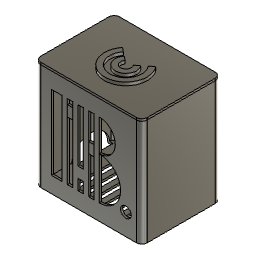
enclosure-lastEdition (Autodesk Fusion 360 design; units mm, degrees)
Autodesk Fusion 360 part; units mm, degrees
note: some values were not read from the file. Chosen so that the rebuilt part matches the saved one: which bodies a step acts on. Set by a fixed rule: which sketch regions a step uses.
sketch "Sketch1" plane through (0, 0, 0) normal (0, 0, 1) x (1, 0, 0)
  line L0 (0, 0) -> (100, 0)
  line L1 (100, 0) -> (100, 74)
  line L2 (100, 74) -> (0, 74)
  line L3 (0, 74) -> (0, 0)
  dimension "d1" = 100
  dimension "d2" = 74
  constraint horizontal L0
  constraint vertical L1
  constraint horizontal L2
  constraint vertical L3
  constraint coincident L0.start L3.end
  measures "d1" distance of L0.start L0.end
  measures "d2" distance of L0.start L2.end
extrude "Extrude1" add sketch "Sketch1" along normal blind 100 makes body 1
fillet "Fillet1" radius 5 1 edges at (100, 0, 50) on bodies 1
fillet "Fillet2" radius 5 1 edges at (0, 0, 50) on bodies 1
fillet "Fillet3" radius 5 1 edges at (100, 74, 50) on bodies 1
fillet "Fillet4" radius 5 1 edges at (0, 74, 50) on bodies 1
shell "Shell1" thickness 2 removed faces 1 at (35, 24.6667, 100) on bodies 1
sketch "Sketch2" plane through (0, 0, 0) normal (-1, 0, 0) x (0, -1, 0)
  line L0 (-69, 100) -> (-69, 0)
  line L1 (-69, 0) -> (-5, 0)
  line L2 (-5, 0) -> (-5, 100)
  line L3 (-5, 100) -> (-69, 100)
  circle A0 centre (-50, 0) radius 18
  dimension "d14" = 36
  constraint coincident L1 A0.centre
  measures "d14" diameter of A0
extrude "Extrude2" cut sketch "Sketch2" against normal blind 5 contours L1 A0 picked at (-55.0244, 4.2742) bodies 1
sketch "Sketch3" plane through (0, 74, 0) normal (0, 1, 0) x (-1, 0, 0)
  line L0 (-5, 0) -> (-5, 100)
  line L1 (-5, 100) -> (-95, 100)
  line L2 (-95, 100) -> (-95, 0)
  line L3 (-95, 0) -> (-5, 0)
  line L4 (-45.9741, 3.8259) -> (-20.9741, 3.8259) construction
  line L5 (-20.9741, 3.8259) -> (-20.9741, 13.8259) construction
  line L6 (-20.9741, 13.8259) -> (-45.9741, 13.8259) construction
  line L7 (-45.9741, 13.8259) -> (-45.9741, 3.8259) construction
  dimension "d17" = 10
  text T0 "CASA" font "Arial" height 10 align left top in box 25 x 10 at (-45.9741, 3.8259) x (1, 0) y (0, 1) spacing 1
extrude "Extrude3" cut sketch "Sketch3" against normal blind 10 text T0 bodies 1 makes body 2 at (13.1683, 72, 8.8554) makes body 3 at (35, 0, 33.3333)
sketch "Sketch4" plane through (0, 0, 0) normal (0, 0, 1) x (1, 0, 0)
sketch "Sketch5" plane through (0, 0, 0) normal (0, 1, 0) x (1, 0, 0)
  line L0 (5, 0) -> (15, 0)
  line L1 (15, -15) -> (25, -15)
  line L2 (25, -15) -> (25, -85)
  line L3 (25, -85) -> (15, -85)
  line L4 (15, -85) -> (15, -15)
  line L5 (30, -15) -> (35, -15)
  line L6 (35, -15) -> (35, -85)
  line L7 (35, -85) -> (30, -85)
  line L8 (30, -85) -> (30, -15)
  line L9 (40, -15) -> (45, -15)
  line L10 (45, -15) -> (45, -85)
  line L11 (45, -85) -> (40, -85)
  line L12 (40, -85) -> (40, -15)
  line L13 (50, -15) -> (55, -15)
  line L14 (55, -15) -> (55, -85)
  line L15 (55, -85) -> (50, -85)
  line L16 (50, -85) -> (50, -15)
  arc A0 (60, -85) -> (60, -55) centre (60, -70) ccw
  arc A1 (60, -55) -> (60, -15) centre (60, -35) ccw
  line L17 (60, -85) -> (60, -15)
  line L18 (40, -25) -> (38, -25)
  line L19 (38, -25) -> (38, -35)
  line L20 (38, -35) -> (40, -35)
  line L21 (40, -35) -> (40, -25)
  line L22 (40, -25) -> (47, -25)
  line L23 (47, -25) -> (47, -35)
  line L24 (47, -35) -> (40, -35)
  line L25 (40, -35) -> (40, -25)
  line L26 (30, -70) -> (28, -70)
  line L27 (28, -80) -> (30, -80)
  line L28 (30, -80) -> (30, -70)
  line L29 (30, -70) -> (37, -70)
  line L30 (37, -80) -> (30, -80)
  line L31 (30, -80) -> (30, -70)
  line L32 (50, -50) -> (48, -50)
  line L33 (48, -50) -> (48, -60)
  line L34 (48, -60) -> (50, -60)
  line L35 (50, -60) -> (50, -50)
  line L36 (48, -50) -> (57, -50)
  line L37 (57, -50) -> (57, -60)
  line L38 (57, -60) -> (48, -60)
  line L39 (48, -60) -> (48, -50)
  dimension "d22" = 2
  dimension "d23" = 10
  dimension "d24" = 7
  dimension "d25" = 10
  dimension "d26" = 2
  dimension "d27" = 7
  dimension "d28" = 2
  dimension "d29" = 9
  dimension "d30" = 10
  constraint horizontal L0
  constraint horizontal L1
  constraint vertical L2
  constraint horizontal L3
  constraint vertical L4
  constraint horizontal L5
  constraint vertical L6
  constraint horizontal L7
  constraint vertical L8
  constraint horizontal L9
  constraint vertical L10
  constraint horizontal L11
  constraint vertical L12
  constraint horizontal L13
  constraint vertical L14
  constraint horizontal L15
  constraint vertical L16
  constraint vertical L17
  constraint horizontal L18
  constraint vertical L19
  constraint horizontal L20
  constraint vertical L21
  constraint coincident L12 L18.start
  constraint horizontal L22
  constraint vertical L23
  constraint horizontal L24
  constraint vertical L25
  constraint horizontal L26
  constraint horizontal L27
  constraint vertical L28
  constraint coincident L8 L26.start
  constraint horizontal L29
  constraint horizontal L30
  constraint vertical L31
  constraint horizontal L32
  constraint vertical L33
  constraint horizontal L34
  constraint vertical L35
  constraint midpoint L16 L32.start
  constraint horizontal L36
  constraint vertical L37
  constraint horizontal L38
  constraint vertical L39
  measures "d22" distance of L18.start L18.end
  measures "d23" distance of L18.start L20.end
  measures "d24" distance of L18.start L22.end
  measures "d25" distance of L18.start L20.end
  measures "d26" distance of L26.start L26.end
  measures "d27" distance of L26.start L29.end
  measures "d28" distance of L32.start L32.end
  measures "d29" distance of L32.end L36.end
  measures "d30" distance of L32.end L33.end
extrude "Extrude5" cut sketch "Sketch5" along normal blind 5 contours L1 L2 L3 L4 bodies 3
extrude "Extrude4" cut sketch "Sketch5" along normal blind 5 contours L1 L2 L3 L4 bodies 3
extrude "Extrude6" cut sketch "Sketch5" along normal blind 5 contours L5 L6 L8 L29 bodies 3
extrude "Extrude7" cut sketch "Sketch5" along normal blind 5 contours L10 L11 L12 L24 bodies 3
extrude "Extrude8" cut sketch "Sketch5" along normal blind 10 contours A1 L17 bodies 3
extrude "Extrude9" cut sketch "Sketch5" along normal blind 5 contours A0 L17 bodies 3
extrude "Extrude10" cut sketch "Sketch5" along normal blind 5 contours L14 L15 L16 L38 bodies 3
extrude "Extrude11" cut sketch "Sketch5" along normal blind 5 contours L13 L14 L16 L36 bodies 3
extrude "Extrude12" cut sketch "Sketch5" along normal blind 5 contours L6 L8 L28 L29 L30 L31 bodies 3
extrude "Extrude13" cut sketch "Sketch5" along normal blind 5 contours L14 L16 L35 L36 L38 bodies 3
extrude "Extrude14" add sketch "Sketch5" along normal blind 2 separate body contours L14 L16 L35 L36 L38 makes body 4
extrude "Extrude15" add sketch "Sketch5" along normal blind 2 separate body contours L6 L8 L28 L29 L30 L31 makes body 5
extrude "Extrude16" cut sketch "Sketch5" along normal blind 2 contours L9 L10 L12 L22 bodies 3
extrude "Extrude17" cut sketch "Sketch5" along normal blind 2 contours L6 L7 L8 L30 bodies 3
sketch "Sketch6" plane through (0, 0, 0) normal (0, -1, 0) x (1, 0, 0)
  line L0 (35, 85) -> (35, 15)
  line L1 (35, 15) -> (30, 15)
  line L2 (30, 15) -> (30, 85)
  line L3 (30, 85) -> (35, 85)
  line L4 (45, 15) -> (40, 15)
  line L5 (40, 15) -> (40, 25)
  line L6 (40, 25) -> (45, 25)
  line L7 (45, 25) -> (45, 15)
  line L8 (50, 15) -> (50, 85)
  line L9 (50, 85) -> (55, 85)
  line L10 (55, 85) -> (55, 15)
  line L11 (55, 15) -> (50, 15)
  line L12 (5, 100) -> (5, 0)
  line L13 (5, 0) -> (95, 0)
  line L14 (95, 0) -> (95, 100)
  line L15 (95, 100) -> (5, 100)
  line L16 (15, 15) -> (15, 85)
  line L17 (15, 85) -> (25, 85)
  line L18 (25, 85) -> (25, 15)
  line L19 (25, 15) -> (15, 15)
  line L20 (45, 85) -> (45, 35)
  line L21 (45, 35) -> (40, 35)
  line L22 (40, 35) -> (40, 85)
  line L23 (40, 85) -> (45, 85)
  line L24 (60, 15) -> (60, 55)
  line L25 (60, 55) -> (60, 85)
  arc A0 (60, 55) -> (60, 85) centre (60, 70) ccw
  arc A1 (60, 15) -> (60, 55) centre (60, 35) ccw
  circle A2 centre (85, 20) radius 5
  dimension "d57" = 10
  measures "d57" diameter of A2
extrude "Extrude18" cut sketch "Sketch6" against normal blind 5 contours A2 bodies 3
sketch "Sketch7" plane through (0, 0, 0) normal (0, 0, 1) x (1, 0, 0)
sketch "Sketch8" plane through (0, 0, 0) normal (0, 0, -1) x (1, 0, 0)
  line L0 (5, -68) -> (0, -68)
  line L1 (0, -68) -> (0, -69)
  arc A0 (0, -69) -> (5, -74) centre (5, -69) ccw
  line L2 (5, -74) -> (95, -74)
  arc A1 (95, -74) -> (100, -69) centre (95, -69) ccw
  line L3 (100, -69) -> (100, -5)
  arc A2 (100, -5) -> (95, 0) centre (95, -5) ccw
  line L4 (95, 0) -> (5, 0)
  arc A3 (5, 0) -> (0, -5) centre (5, -5) ccw
  line L5 (0, -5) -> (0, -32)
  line L6 (0, -32) -> (5, -32)
  line L7 (5, -32) -> (5, -68)
  line L8 (20, -10) -> (25, -10)
  line L9 (25, -10) -> (25, -65)
  line L10 (25, -65) -> (20, -65)
  line L11 (20, -65) -> (20, -10)
  line L12 (30, -10) -> (35, -10)
  line L13 (35, -10) -> (35, -65)
  line L14 (35, -65) -> (30, -65)
  line L15 (30, -65) -> (30, -10)
  line L16 (40, -10) -> (45, -10)
  line L17 (45, -10) -> (45, -65)
  line L18 (45, -65) -> (40, -65)
  line L19 (40, -65) -> (40, -10)
  line L20 (50, -10) -> (55, -10)
  line L21 (55, -10) -> (55, -65)
  line L22 (55, -65) -> (50, -65)
  line L23 (50, -65) -> (50, -10)
  line L24 (60, -10) -> (65, -10)
  line L25 (65, -10) -> (65, -65)
  line L26 (65, -65) -> (60, -65)
  line L27 (60, -65) -> (60, -10)
  line L28 (70, -10) -> (75, -10)
  line L29 (75, -10) -> (75, -65)
  line L30 (75, -65) -> (70, -65)
  line L31 (70, -65) -> (70, -10)
  line L32 (80, -10) -> (85, -10)
  line L33 (85, -10) -> (85, -65)
  line L34 (85, -65) -> (80, -65)
  line L35 (80, -65) -> (80, -10)
  constraint horizontal L8
  constraint vertical L9
  constraint horizontal L10
  constraint vertical L11
  constraint horizontal L12
  constraint vertical L13
  constraint horizontal L14
  constraint vertical L15
  constraint horizontal L16
  constraint vertical L17
  constraint horizontal L18
  constraint vertical L19
  constraint horizontal L20
  constraint vertical L21
  constraint horizontal L22
  constraint vertical L23
  constraint horizontal L24
  constraint vertical L25
  constraint horizontal L26
  constraint vertical L27
  constraint horizontal L28
  constraint vertical L29
  constraint horizontal L30
  constraint vertical L31
  constraint horizontal L32
  constraint vertical L33
  constraint horizontal L34
  constraint vertical L35
extrude "Extrude19" cut sketch "Sketch8" against normal blind 10 contours L8 L9 L10 L11 bodies 3
extrude "Extrude20" cut sketch "Sketch8" against normal blind 10 contours L12 L13 L14 L15 bodies 3
extrude "Extrude21" cut sketch "Sketch8" against normal blind 10 contours L16 L17 L18 L19 bodies 3
extrude "Extrude22" cut sketch "Sketch8" against normal blind 5 contours L20 L21 L22 L23 bodies 3
extrude "Extrude23" cut sketch "Sketch8" against normal blind 5 contours L24 L25 L26 L27 bodies 3
extrude "Extrude24" cut sketch "Sketch8" against normal blind 10 contours L28 L29 L30 L31 bodies 3
extrude "Extrude25" cut sketch "Sketch8" against normal blind 5 contours L32 L33 L34 L35 bodies 3
sketch "Sketch9" plane through (0, 74, 0) normal (0, 1, 0) x (-1, 0, 0)
  line L0 (-34.0982, 6.8545) -> (-35.1965, 3.8259)
  line L1 (-35.1965, 3.8259) -> (-36.6017, 3.8259)
  line L2 (-36.6017, 3.8259) -> (-32.7613, 13.8259)
  line L3 (-32.7613, 13.8259) -> (-31.3356, 13.8259)
  line L4 (-31.3356, 13.8259) -> (-27.2429, 3.8259)
  line L5 (-27.2429, 3.8259) -> (-28.7504, 3.8259)
  line L6 (-28.7504, 3.8259) -> (-29.9168, 6.8545)
  line L7 (-29.9168, 6.8545) -> (-34.0982, 6.8545)
  spline S0 degree 3 poles (-24.6508, 4.051) (-24.9381, 4.1976) (-25.5056, 4.4873) (-25.8969, 4.9898) (-26.0901, 5.2379) knots 0 0 0 0 0.095489 0.188591 0.188591 0.188591 0.188591
  spline S1 degree 3 poles (-26.0901, 5.2379) (-26.2425, 5.5147) (-26.5516, 6.0762) (-26.6074, 6.7149) (-26.6358, 7.0387) knots 0 0 0 0 0.093688 0.190021 0.190021 0.190021 0.190021
  line L8 (-26.6358, 7.0387) -> (-25.3875, 7.1478)
  spline S2 degree 3 poles (-25.3875, 7.1478) (-25.3523, 6.9152) (-25.2865, 6.4796) (-25.0762, 6.0932) (-24.9782, 5.9132) knots 0 0 0 0 0.069938 0.130961 0.130961 0.130961 0.130961
  spline S3 degree 3 poles (-24.9782, 5.9132) (-24.8475, 5.7586) (-24.5676, 5.4273) (-24.177, 5.237) (-23.9686, 5.1356) knots 0 0 0 0 0.060063 0.128681 0.128681 0.128681 0.128681
  spline S4 degree 3 poles (-23.9686, 5.1356) (-23.7294, 5.0501) (-23.2333, 4.8727) (-22.7066, 4.8526) (-22.4339, 4.8423) knots 0 0 0 0 0.075741 0.157075 0.157075 0.157075 0.157075
  spline S5 degree 3 poles (-22.4339, 4.8423) (-22.1943, 4.8496) (-21.738, 4.8636) (-21.3033, 5.0017) (-21.0969, 5.0674) knots 0 0 0 0 0.071504 0.136162 0.136162 0.136162 0.136162
  spline S6 degree 3 poles (-21.0969, 5.0674) (-20.9199, 5.1441) (-20.5889, 5.2878) (-20.3491, 5.5563) (-20.2374, 5.6813) knots 0 0 0 0 0.057059 0.106742 0.106742 0.106742 0.106742
  spline S7 degree 3 poles (-20.2374, 5.6813) (-20.1538, 5.8149) (-19.989, 6.0784) (-19.9635, 6.3881) (-19.9509, 6.5408) knots 0 0 0 0 0.046527 0.091777 0.091777 0.091777 0.091777
  spline S8 degree 3 poles (-19.9509, 6.5408) (-19.9615, 6.6915) (-19.9823, 6.988) (-20.1442, 7.2369) (-20.2238, 7.3593) knots 0 0 0 0 0.044523 0.087558 0.087558 0.087558 0.087558
  spline S9 degree 3 poles (-20.2238, 7.3593) (-20.3387, 7.476) (-20.5959, 7.737) (-20.9361, 7.876) (-21.1242, 7.9528) knots 0 0 0 0 0.048661 0.108834 0.108834 0.108834 0.108834
  spline S10 degree 3 poles (-21.1242, 7.9528) (-21.339, 8.0214) (-21.9252, 8.2087) (-22.5247, 8.3485) (-22.9045, 8.4371) knots 0 0 0 0 0.067641 0.184566 0.184566 0.184566 0.184566
  spline S11 degree 3 poles (-22.9045, 8.4371) (-23.2993, 8.5324) (-23.9596, 8.6918) (-24.5839, 8.9577) (-24.8349, 9.0646) knots 0 0 0 0 0.121554 0.203286 0.203286 0.203286 0.203286
  spline S12 degree 3 poles (-24.8349, 9.0646) (-25.0549, 9.1915) (-25.4722, 9.4322) (-25.7667, 9.8125) (-25.9059, 9.9923) knots 0 0 0 0 0.075345 0.142899 0.142899 0.142899 0.142899
  spline S13 degree 3 poles (-25.9059, 9.9923) (-26.0074, 10.1855) (-26.2127, 10.5765) (-26.24, 11.0175) (-26.2538, 11.2406) knots 0 0 0 0 0.064671 0.1309 0.1309 0.1309 0.1309
  spline S14 degree 3 poles (-26.2538, 11.2406) (-26.2352, 11.4897) (-26.1978, 11.9924) (-25.9494, 12.4312) (-25.824, 12.6526) knots 0 0 0 0 0.073943 0.149233 0.149233 0.149233 0.149233
  spline S15 degree 3 poles (-25.824, 12.6526) (-25.66, 12.8616) (-25.3207, 13.2937) (-24.825, 13.5322) (-24.5689, 13.6554) knots 0 0 0 0 0.078589 0.162564 0.162564 0.162564 0.162564
  spline S16 degree 3 poles (-24.5689, 13.6554) (-24.2811, 13.7548) (-23.6868, 13.9602) (-23.0582, 13.9841) (-22.734, 13.9964) knots 0 0 0 0 0.090819 0.187546 0.187546 0.187546 0.187546
  spline S17 degree 3 poles (-22.734, 13.9964) (-22.3821, 13.9845) (-21.7109, 13.9618) (-21.0776, 13.7403) (-20.7763, 13.6349) knots 0 0 0 0 0.104926 0.200105 0.200105 0.200105 0.200105
  spline S18 degree 3 poles (-20.7763, 13.6349) (-20.5108, 13.5058) (-19.9942, 13.2546) (-19.6392, 12.8037) (-19.4666, 12.5844) knots 0 0 0 0 0.087276 0.169846 0.169846 0.169846 0.169846
  spline S19 degree 3 poles (-19.4666, 12.5844) (-19.3318, 12.3427) (-19.0581, 11.852) (-19.0033, 11.2926) (-18.9755, 11.0087) knots 0 0 0 0 0.082079 0.166634 0.166634 0.166634 0.166634
  line L9 (-18.9755, 11.0087) -> (-20.2442, 10.9132)
  spline S20 degree 3 poles (-20.2442, 10.9132) (-20.2921, 11.2042) (-20.3824, 11.7527) (-20.7619, 12.1562) (-20.94, 12.3457) knots 0 0 0 0 0.08621 0.16249 0.16249 0.16249 0.16249
  spline S21 degree 3 poles (-20.94, 12.3457) (-21.1768, 12.4865) (-21.71, 12.8035) (-22.3331, 12.8205) (-22.6794, 12.83) knots 0 0 0 0 0.081374 0.183222 0.183222 0.183222 0.183222
  spline S22 degree 3 poles (-22.6794, 12.83) (-23.0343, 12.8244) (-23.657, 12.8145) (-24.1993, 12.5153) (-24.4325, 12.3866) knots 0 0 0 0 0.104444 0.183256 0.183256 0.183256 0.183256
  spline S23 degree 3 poles (-24.4325, 12.3866) (-24.5916, 12.2372) (-24.8992, 11.9483) (-24.9525, 11.5309) (-24.9782, 11.3293) knots 0 0 0 0 0.063278 0.122345 0.122345 0.122345 0.122345
  spline S24 degree 3 poles (-24.9782, 11.3293) (-24.9626, 11.1582) (-24.9317, 10.8191) (-24.7028, 10.5673) (-24.5894, 10.4425) knots 0 0 0 0 0.050066 0.099215 0.099215 0.099215 0.099215
  spline S25 degree 3 poles (-24.5894, 10.4425) (-24.3632, 10.3161) (-23.7417, 9.9686) (-23.0424, 9.8205) (-22.5976, 9.7263) knots 0 0 0 0 0.077412 0.212667 0.212667 0.212667 0.212667
  spline S26 degree 3 poles (-22.5976, 9.7263) (-22.1398, 9.6252) (-21.3874, 9.4591) (-20.664, 9.1953) (-20.3806, 9.0919) knots 0 0 0 0 0.140418 0.230805 0.230805 0.230805 0.230805
  spline S27 degree 3 poles (-20.3806, 9.0919) (-20.1141, 8.9564) (-19.6141, 8.7022) (-19.2578, 8.2704) (-19.0914, 8.0687) knots 0 0 0 0 0.088586 0.166163 0.166163 0.166163 0.166163
  spline S28 degree 3 poles (-19.0914, 8.0687) (-18.9701, 7.8533) (-18.722, 7.4129) (-18.6911, 6.9079) (-18.6753, 6.6499) knots 0 0 0 0 0.073157 0.149584 0.149584 0.149584 0.149584
  spline S29 degree 3 poles (-18.6753, 6.6499) (-18.6955, 6.3859) (-18.7364, 5.8498) (-18.9991, 5.3805) (-19.1324, 5.1424) knots 0 0 0 0 0.078429 0.159219 0.159219 0.159219 0.159219
  spline S30 degree 3 poles (-19.1324, 5.1424) (-19.3058, 4.919) (-19.6642, 4.4575) (-20.1818, 4.1849) (-20.4489, 4.0442) knots 0 0 0 0 0.083824 0.173212 0.173212 0.173212 0.173212
  spline S31 degree 3 poles (-20.4489, 4.0442) (-20.7479, 3.9308) (-21.3675, 3.696) (-22.0299, 3.6692) (-22.3725, 3.6554) knots 0 0 0 0 0.095294 0.197395 0.197395 0.197395 0.197395
  spline S32 degree 3 poles (-22.3725, 3.6554) (-22.7926, 3.6661) (-23.5724, 3.686) (-24.3104, 3.9358) (-24.6508, 4.051) knots 0 0 0 0 0.125221 0.232411 0.232411 0.232411 0.232411
  line L10 (-15.4625, 6.8545) -> (-16.5607, 3.8259)
  line L11 (-16.5607, 3.8259) -> (-17.9659, 3.8259)
  line L12 (-17.9659, 3.8259) -> (-14.1255, 13.8259)
  line L13 (-14.1255, 13.8259) -> (-12.6999, 13.8259)
  line L14 (-12.6999, 13.8259) -> (-8.6071, 3.8259)
  line L15 (-8.6071, 3.8259) -> (-10.1146, 3.8259)
  line L16 (-10.1146, 3.8259) -> (-11.2811, 6.8545)
  line L17 (-11.2811, 6.8545) -> (-15.4625, 6.8545)
  spline S33 degree 3 poles (-41.3834, 4.7877) (-41.0308, 4.8112) (-40.3451, 4.8571) (-39.7768, 5.2419) (-39.5007, 5.4289) knots 0 0 0 0 0.103904 0.202094 0.202094 0.202094 0.202094
  spline S34 degree 3 poles (-39.5007, 5.4289) (-39.262, 5.6812) (-38.7496, 6.2229) (-38.5589, 6.9459) (-38.457, 7.332) knots 0 0 0 0 0.102565 0.220156 0.220156 0.220156 0.220156
  line L18 (-38.457, 7.332) -> (-37.1337, 6.9978)
  spline S35 degree 3 poles (-37.1337, 6.9978) (-37.2898, 6.495) (-37.5865, 5.5399) (-38.2976, 4.8397) (-38.6344, 4.508) knots 0 0 0 0 0.155139 0.294739 0.294739 0.294739 0.294739
  spline S36 degree 3 poles (-38.6344, 4.508) (-39.0223, 4.2594) (-39.8261, 3.7443) (-40.7805, 3.6857) (-41.2742, 3.6554) knots 0 0 0 0 0.135874 0.281542 0.281542 0.281542 0.281542
  spline S37 degree 3 poles (-41.2742, 3.6554) (-41.7727, 3.6732) (-42.6985, 3.7065) (-43.5255, 4.1195) (-43.9073, 4.3102) knots 0 0 0 0 0.147568 0.27413 0.27413 0.27413 0.27413
  spline S38 degree 3 poles (-43.9073, 4.3102) (-44.2264, 4.5613) (-44.8853, 5.0798) (-45.2572, 5.8322) (-45.4489, 6.2202) knots 0 0 0 0 0.120241 0.248224 0.248224 0.248224 0.248224
  spline S39 degree 3 poles (-45.4489, 6.2202) (-45.602, 6.6473) (-45.9129, 7.5141) (-45.9535, 8.4342) (-45.9741, 8.9009) knots 0 0 0 0 0.135296 0.274559 0.274559 0.274559 0.274559
  spline S40 degree 3 poles (-45.9741, 8.9009) (-45.9544, 9.3947) (-45.9167, 10.3378) (-45.5536, 11.208) (-45.3807, 11.6226) knots 0 0 0 0 0.146897 0.280549 0.280549 0.280549 0.280549
  spline S41 degree 3 poles (-45.3807, 11.6226) (-45.1622, 11.9865) (-44.7306, 12.7054) (-44.0287, 13.1633) (-43.6822, 13.3893) knots 0 0 0 0 0.125527 0.247938 0.247938 0.247938 0.247938
  spline S42 degree 3 poles (-43.6822, 13.3893) (-43.302, 13.5664) (-42.5319, 13.9251) (-41.6834, 13.9724) (-41.2538, 13.9964) knots 0 0 0 0 0.124581 0.252361 0.252361 0.252361 0.252361
  spline S43 degree 3 poles (-41.2538, 13.9964) (-40.7816, 13.9705) (-39.8767, 13.9208) (-39.1009, 13.4551) (-38.7299, 13.2324) knots 0 0 0 0 0.139445 0.267264 0.267264 0.267264 0.267264
  spline S44 degree 3 poles (-38.7299, 13.2324) (-38.4127, 12.9448) (-37.7567, 12.3499) (-37.4583, 11.5149) (-37.3043, 11.0837) knots 0 0 0 0 0.126424 0.261432 0.261432 0.261432 0.261432
  line L19 (-37.3043, 11.0837) -> (-38.6071, 10.7768)
  spline S45 degree 3 poles (-38.6071, 10.7768) (-38.7251, 11.1069) (-38.9422, 11.7148) (-39.4052, 12.1619) (-39.6167, 12.3661) knots 0 0 0 0 0.103493 0.190549 0.190549 0.190549 0.190549
  spline S46 degree 3 poles (-39.6167, 12.3661) (-39.8593, 12.5113) (-40.3709, 12.8173) (-40.9674, 12.848) (-41.2811, 12.8641) knots 0 0 0 0 0.083509 0.176096 0.176096 0.176096 0.176096
  spline S47 degree 3 poles (-41.2811, 12.8641) (-41.6423, 12.8461) (-42.33, 12.8119) (-42.9278, 12.4726) (-43.2115, 12.3116) knots 0 0 0 0 0.106797 0.203291 0.203291 0.203291 0.203291
  spline S48 degree 3 poles (-43.2115, 12.3116) (-43.4499, 12.1099) (-43.9318, 11.7023) (-44.1738, 11.1191) (-44.2961, 10.8245) knots 0 0 0 0 0.092249 0.186438 0.186438 0.186438 0.186438
  spline S49 degree 3 poles (-44.2961, 10.8245) (-44.3876, 10.5123) (-44.5711, 9.8863) (-44.5969, 9.2345) (-44.6098, 8.9077) knots 0 0 0 0 0.097196 0.194886 0.194886 0.194886 0.194886
  spline S50 degree 3 poles (-44.6098, 8.9077) (-44.5983, 8.506) (-44.5763, 7.7453) (-44.3488, 7.0196) (-44.2415, 6.6772) knots 0 0 0 0 0.119897 0.227033 0.227033 0.227033 0.227033
  spline S51 degree 3 poles (-44.2415, 6.6772) (-44.1034, 6.3835) (-43.8352, 5.8129) (-43.328, 5.4395) (-43.0819, 5.2584) knots 0 0 0 0 0.09565 0.185841 0.185841 0.185841 0.185841
  spline S52 degree 3 poles (-43.0819, 5.2584) (-42.815, 5.1211) (-42.2814, 4.8466) (-41.6827, 4.8073) (-41.3834, 4.7877) knots 0 0 0 0 0.088986 0.177933 0.177933 0.177933 0.177933
  line L20 (-5, 0) -> (-5, 100)
  line L21 (-5, 100) -> (-95, 100)
  line L22 (-95, 100) -> (-95, 0)
  line L23 (-95, 0) -> (-5, 0)
  circle A0 centre (-50, 40) radius 15
  circle A1 centre (-50, 40) radius 20
  circle A2 centre (-50, 80) radius 15
  circle A3 centre (-50, 80) radius 10
  circle A4 centre (-50, 40) radius 5
  circle A5 centre (-50, 40) radius 10
  line L24 (-50, 40) -> (-66.9856, 29.4412)
  line L25 (-50, 40) -> (-32.6922, 29.978)
  constraint concentric A0 A1
  constraint concentric A2 A3
  constraint concentric A1 A4
  constraint concentric A4 A5
  constraint coincident A0.centre A1.centre
  constraint coincident A1 L24.end
  constraint coincident A1 L25.end
extrude "Extrude26" cut sketch "Sketch9" against normal blind 20 contours A0 A1 L24 L25 picked at (-67.8981, 36.2488) bodies 3
extrude "Extrude27" cut sketch "Sketch9" against normal blind 10 contours A4 A5 L24 L25 picked at (-53.5463, 47.5169) bodies 3
sketch "Sketch10" plane through (0, 0, 100) normal (0, 0, 1) x (-1, 0, 0)
  arc A0 (-2, -5) -> (-5, -2) centre (-5, -5) ccw
  line L0 (-2, -5) -> (-2, -69)
  arc A1 (-5, -72) -> (-2, -69) centre (-5, -69) ccw
  line L1 (-5, -72) -> (-95, -72)
  arc A2 (-98, -69) -> (-95, -72) centre (-95, -69) ccw
  line L2 (-98, -69) -> (-98, -5)
  arc A3 (-95, -2) -> (-98, -5) centre (-95, -5) ccw
  line L3 (-95, -2) -> (-5, -2)
  arc A4 (-5, -74) -> (0, -69) centre (-5, -69) ccw
  line L4 (0, -69) -> (0, -5)
  arc A5 (0, -5) -> (-5, 0) centre (-5, -5) ccw
  line L5 (-5, 0) -> (-95, 0)
  arc A6 (-95, 0) -> (-100, -5) centre (-95, -5) ccw
  line L6 (-100, -5) -> (-100, -69)
  arc A7 (-100, -69) -> (-95, -74) centre (-95, -69) ccw
  line L7 (-95, -74) -> (-5, -74)
  line L8 (-125, 0) -> (-225, 0)
  line L9 (-225, 0) -> (-225, -74)
  line L10 (-225, -74) -> (-125, -74)
  line L11 (-125, -74) -> (-125, 0)
  dimension "d78" = 100
  dimension "d79" = 74
  constraint horizontal L8
  constraint vertical L9
  constraint horizontal L10
  constraint vertical L11
  measures "d78" distance of L8.start L8.end
  measures "d79" distance of L8.start L10.end
extrude "Extrude28" add sketch "Sketch10" along normal blind 2 separate body contours L8 L9 L10 L11 makes body 6
fillet "Fillet5" radius 5 1 edges at (225, 0, 101) on bodies 6
fillet "Fillet6" radius 5 1 edges at (225, 74, 101) on bodies 6
fillet "Fillet7" radius 5 1 edges at (125, 0, 101) on bodies 6
fillet "Fillet8" radius 5 1 edges at (125, 74, 101) on bodies 6
sketch "Sketch11" plane through (0, 0, 102) normal (0, 0, 1) x (-1, 0, 0)
  arc A0 (-130, -74) -> (-125, -69) centre (-130, -69) ccw
  line L0 (-125, -69) -> (-125, -5)
  arc A1 (-125, -5) -> (-130, 0) centre (-130, -5) ccw
  line L1 (-130, 0) -> (-220, 0)
  arc A2 (-220, 0) -> (-225, -5) centre (-220, -5) ccw
  line L2 (-225, -5) -> (-225, -69)
  arc A3 (-225, -69) -> (-220, -74) centre (-220, -69) ccw
  line L3 (-220, -74) -> (-130, -74)
  line L4 (-127, -69) -> (-127, -5)
  arc A4 (-127, -5) -> (-130, -2) centre (-130, -5) ccw
  line L5 (-130, -2) -> (-220, -2)
  arc A5 (-220, -2) -> (-223, -5) centre (-220, -5) ccw
  line L6 (-223, -5) -> (-223, -69)
  arc A6 (-223, -69) -> (-220, -72) centre (-220, -69) ccw
  line L7 (-220, -72) -> (-130, -72)
  arc A7 (-130, -72) -> (-127, -69) centre (-130, -69) ccw
  line L8 (-130, -69) -> (-130, -5)
  line L9 (-130, -5) -> (-220, -5)
  line L10 (-220, -5) -> (-220, -69)
  line L11 (-220, -69) -> (-130, -69)
  dimension "d90" = -2
  dimension "d91" = -5
extrude "Extrude29" add sketch "Sketch11" along normal blind 4 contours L4 A4 L5 A5 L6 A6 L7 A7 bodies 6
sketch "Sketch12" plane through (0, 0, 102) normal (0, 0, 1) x (-1, 0, 0)
  line L0 (-130, -69) -> (-130, -5)
  line L1 (-130, -5) -> (-220, -5)
  line L2 (-220, -5) -> (-220, -69)
  line L3 (-220, -69) -> (-130, -69)
sketch "Sketch13" plane through (0, 0, 100) normal (0, 0, -1) x (1, 0, 0)
  arc A0 (125, -69) -> (130, -74) centre (130, -69) ccw
  line L0 (130, -74) -> (220, -74)
  arc A1 (220, -74) -> (225, -69) centre (220, -69) ccw
  line L1 (225, -69) -> (225, -5)
  arc A2 (225, -5) -> (220, 0) centre (220, -5) ccw
  line L2 (220, 0) -> (130, 0)
  arc A3 (130, 0) -> (125, -5) centre (130, -5) ccw
  line L3 (125, -5) -> (125, -69)
  circle A4 centre (175, -35) radius 20
  circle A5 centre (175, -35) radius 15
  circle A6 centre (175, -35) radius 10
  circle A7 centre (175, -35) radius 5
  line L4 (175, -35) -> (150, -55)
  line L5 (150, -55) -> (175, -35)
  line L6 (175, -35) -> (200, -55)
  dimension "d94" = 40
  constraint concentric A4 A5
  constraint concentric A5 A6
  constraint concentric A4 A7
  constraint coincident A4.centre A5.centre
  constraint parallel L4 L5
  measures "d94" diameter of A4
extrude "Extrude30" add sketch "Sketch13" along normal blind 3 contours A6 A7 L4 L5 L6 picked at (177.5233, -27.0805) bodies 6
extrude "Extrude31" add sketch "Sketch13" along normal blind 3 contours A4 A5 L4 L5 L6 picked at (168.0352, -18.0905) bodies 6
move_body "Move1" bodies 6 to x (-1, 0, 0) y (0, 1, 0) z (0, 0, -1) at (250, 0, 194)
move_body "Move2" bodies 6 to x (1, 0, 0) y (0, 1, 0) z (0, 0, 1) at (-25, 0, 10)
move_body "Move3" bodies 6 to x (1, 0, 0) y (0, 1, 0) z (0, 0, 1) at (0, 0, -2)
